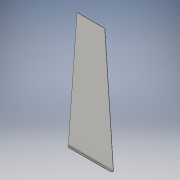
# Autodesk Inventor part: robot side
Saved by Autodesk Inventor 2016 (Build 200138000, 138)
## iProperties
Created: 2017-03-16
Part Number: robot side
Material: Generic
Document SubType Name: Sheet Metal
Designer: earlyp
Density: 1 g/cm^3
Sheet Metal Rule: Default
Appearance: Default
Author: earlyp
Autodesk Inventor part; units mm, degrees
ref_plane "YZ Plane" through (0, 0, 0) normal (1, 0, 0) x (0, 1, 0)
ref_plane "XZ Plane" through (0, 0, 0) normal (0, 1, 0) x (-1, 0, 0)
ref_plane "XY Plane" through (0, 0, 0) normal (0, 0, 1) x (1, 0, 0)
sketch "Sketch1" plane through (0, 0, 0) normal (0, 0, 1) x (1, 0, 0)
  line L0 (-254, 0) -> (254, 0)
  line L1 (-156.845, 1347.6224) -> (156.845, 1347.6224)
  line L2 (-156.845, 1347.6224) -> (-254, 0)
  line L3 (254, 0) -> (156.845, 1347.6224)
  point P0 (0, 0)
  point P1 (0, 0)
  point P2 (0, 1347.6224)
  dimension "d0" = 508
  dimension "d1" = 313.69
  dimension "d2" = 1347.6224
  measures "d0" distance of L0.start L0.end
  measures "d1" distance of L1.start L1.end
  measures "d2" vertical distance of L0.end L1.end
extrude "Plate1" add sketch "Sketch1" along normal blind 3.175
sketch "Sketch3" plane through (254, -3.1268, 6.9013) normal (0, -0.9848078, 0.1736482) x (1, 0, 0)
  line L0 (-508, 0) -> (0, 0)
  line L1 (0, 0) -> (0, 17.8324)
  line L2 (0, 17.8324) -> (-508, 17.8324)
  line L3 (-508, 17.8324) -> (-508, 0)
  constraints: 6 end point, 1 horizontal, 1 perpendicular, 1 vertical
edge flange "Flange2" height 25.4 angle 100 thickness 3.175 bend radius 3.175 thickness toward (0, -0.9848078, 0.1736482) relief tear relief width 3.175 relief depth 1.5875 edges at (0, 0, 3.175) wall of the first edge with corners at (-254, -3.1268, 6.9013) (254, -3.1268, 6.9013) (254, -0.0302, 24.4628) (-254, -0.0302, 24.4628)
bend "Bend2"
corner "Corner2"
sketch "Sketch4" plane through (-254, -0.0302, 24.4628) normal (0, 0.9848078, -0.1736482) x (1, 0, 0)
  line L0 (508, 17.8324) -> (0, 17.8324) projected
  line L1 (508, 17.8324) -> (487.7938, 0)
  line L2 (0, 0) -> (508, 0) projected
  line L3 (487.7938, 0) -> (508, 0)
  line L4 (508, 0) -> (508, 17.8324) projected
  line L5 (508, 0) -> (508, 17.8324)
  line L6 (508, 17.8324) -> (487.7938, 0)
  point P0 (254, 24.0859)
  constraints: 8 end point, 3 point on line, 2 collinear, 1 perpendicular
extrude "Cut1" cut sketch "Sketch4" against normal blind 3.175
sketch "Sketch5" plane through (-254, -3.1268, 6.9013) normal (0, 0.9848078, -0.1736482) x (1, 0, 0)
  line L0 (0, -17.8324) -> (0, 0) projected
  line L1 (0, 0) -> (20.2032, -17.8324)
  line L2 (0, -17.8324) -> (487.7938, -17.8324) projected
  point P0 (254, 6.2535)
  constraints: 2 end point, 1 point on line
extrude "Cut2" cut sketch "Sketch5" against normal blind 3.175
equation "\"d24\" = Thickness"
equation "\"d26\" = Thickness"
equation "\"d14\" = BendReliefWidth"
equation "\"d15\" = BendReliefDepth"
equation "\"d16\" = MinimumRemnant"
equation "\"d17\" = BendRadius"
equation "\"d20\" = BendRadius"
equation "\"d21\" = CornerReliefSize"
equation "\"d22\" = GapSize"
equation "\"d23\" = JacobiRadiusSize"
equation "\"BendRadius\" = Thickness"
equation "\"BendReliefWidth\" = Thickness"
equation "\"BendReliefDepth\" = 0.5 * Thickness"
equation "\"CornerReliefSize\" = 4 * Thickness"
equation "\"MinimumRemnant\" = 2 * Thickness"
equation "\"TransitionRadius\" = BendRadius"
equation "\"JacobiRadiusSize\" = BendRadius"
equation "\"GapSize\" = Thickness"
equation "\"d3\" = BendRadius"
equation "\"Thickness\" = 3.175"
body "Solid1"
